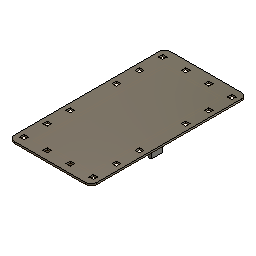
12 V Battery Holder (Autodesk Fusion 360 design; units mm, degrees)
Autodesk Fusion 360 part; units mm, degrees
note: some values were not read from the file. Set by a fixed rule: which sketch regions a step uses.
sketch "Sketch1" plane through (0, 0, 0) normal (0, 1, 0) x (1, 0, 0)
  line L0 (0, 0) -> (58.7375, 0)
  line L1 (58.7375, 0) -> (58.7375, -139.7)
  line L2 (58.7375, -139.7) -> (0, -139.7)
  line L3 (0, -139.7) -> (0, 0)
  line L4 (61.2775, -142.24) -> (-2.54, -142.24)
  line L5 (-2.54, -142.24) -> (-2.54, 2.54)
  line L6 (-2.54, 2.54) -> (61.2775, 2.54)
  line L7 (61.2775, 2.54) -> (61.2775, -142.24)
  line L8 (29.3688, 0) -> (29.3688, -139.7) construction
  line L9 (-8.7313, 6.35) -> (67.4687, 6.35) construction
  line L10 (67.4687, 6.35) -> (67.4688, -146.05)
  line L11 (67.4688, -146.05) -> (-8.7313, -146.05) construction
  line L12 (-8.7313, -146.05) -> (-8.7313, 6.35) construction
  line L13 (-8.7313, 6.35) -> (67.4688, -146.05) construction
  line L14 (67.4687, 6.35) -> (-8.7313, -146.05) construction
  line L15 (-11.1443, 8.763) -> (-6.3183, 8.763)
  line L16 (-6.3183, 8.763) -> (-6.3183, 3.937)
  line L17 (-6.3183, 3.937) -> (-11.1443, 3.937)
  line L18 (-11.1443, 3.937) -> (-11.1443, 8.763)
  line L19 (-11.1443, 8.763) -> (-6.3183, 3.937) construction
  line L20 (-6.3183, 8.763) -> (-11.1443, 3.937) construction
  line L21 (19.0817, 8.763) -> (19.0817, 3.937)
  line L22 (19.0817, 3.937) -> (14.2557, 3.937)
  line L23 (14.2557, 3.937) -> (14.2557, 8.763)
  line L24 (14.2557, 8.763) -> (19.0817, 8.763)
  line L25 (44.4817, 8.763) -> (44.4817, 3.937)
  line L26 (44.4817, 3.937) -> (39.6557, 3.937)
  line L27 (39.6557, 3.937) -> (39.6557, 8.763)
  line L28 (39.6557, 8.763) -> (44.4817, 8.763)
  line L29 (-6.3183, -143.637) -> (-6.3183, -148.463)
  line L30 (-6.3183, -148.463) -> (-11.1443, -148.463)
  line L31 (-11.1443, -148.463) -> (-11.1443, -143.637)
  line L32 (-11.1443, -143.637) -> (-6.3183, -143.637)
  line L33 (19.0817, -143.637) -> (19.0817, -148.463)
  line L34 (19.0817, -148.463) -> (14.2557, -148.463)
  line L35 (14.2557, -148.463) -> (14.2557, -143.637)
  line L36 (14.2557, -143.637) -> (19.0817, -143.637)
  line L37 (44.4817, -143.637) -> (44.4817, -148.463)
  line L38 (44.4817, -148.463) -> (39.6557, -148.463)
  line L39 (39.6557, -148.463) -> (39.6557, -143.637)
  line L40 (39.6557, -143.637) -> (44.4817, -143.637)
  line L41 (69.8817, 8.763) -> (69.8817, 3.937)
  line L42 (69.8817, 3.937) -> (65.0557, 3.937)
  line L43 (65.0557, 3.937) -> (65.0557, 8.763)
  line L44 (65.0557, 8.763) -> (69.8817, 8.763)
  line L45 (69.8817, -143.637) -> (69.8817, -148.463)
  line L46 (69.8817, -148.463) -> (65.0557, -148.463)
  line L47 (65.0557, -148.463) -> (65.0557, -143.637)
  line L48 (65.0557, -143.637) -> (69.8817, -143.637)
  line L49 (74.6125, -155.575) -> (-15.875, -155.575)
  line L50 (-15.875, -155.575) -> (-15.875, 15.875)
  line L51 (-15.875, 15.875) -> (74.6125, 15.875)
  line L52 (74.6125, 15.875) -> (74.6125, -155.575)
  line L53 (58.7375, -125.73) -> (61.2775, -125.73)
  line L54 (61.2775, -125.73) -> (61.2775, -119.38)
  line L55 (61.2775, -119.38) -> (58.7375, -119.38)
  line L56 (58.7375, -119.38) -> (58.7375, -125.73)
  line L57 (60.0075, -125.73) -> (60.0075, -119.38)
  line L58 (29.3688, -69.85) -> (58.7375, -69.85) construction
  line L59 (61.2775, -20.32) -> (58.7375, -20.32)
  line L60 (58.7375, -20.32) -> (58.7375, -13.97)
  line L61 (58.7375, -13.97) -> (61.2775, -13.97)
  line L62 (61.2775, -13.97) -> (61.2775, -20.32)
  line L63 (-11.1443, -21.463) -> (-11.1443, -16.637)
  line L64 (-6.3183, -21.463) -> (-11.1443, -21.463)
  line L65 (-6.3183, -16.637) -> (-6.3183, -21.463)
  line L66 (-11.1443, -16.637) -> (-6.3183, -16.637)
  line L67 (69.8817, -21.463) -> (65.0557, -21.463)
  line L68 (69.8817, -16.637) -> (69.8817, -21.463)
  line L69 (65.0557, -21.463) -> (65.0557, -16.637)
  line L70 (65.0557, -16.637) -> (69.8817, -16.637)
  line L71 (-11.1443, -46.863) -> (-11.1443, -42.037)
  line L72 (-6.3183, -46.863) -> (-11.1443, -46.863)
  line L73 (-6.3183, -42.037) -> (-6.3183, -46.863)
  line L74 (-11.1443, -42.037) -> (-6.3183, -42.037)
  line L75 (69.8817, -46.863) -> (65.0557, -46.863)
  line L76 (69.8817, -42.037) -> (69.8817, -46.863)
  line L77 (65.0557, -46.863) -> (65.0557, -42.037)
  line L78 (65.0557, -42.037) -> (69.8817, -42.037)
  line L79 (-11.1443, -72.263) -> (-11.1443, -67.437)
  line L80 (-6.3183, -72.263) -> (-11.1443, -72.263)
  line L81 (-6.3183, -67.437) -> (-6.3183, -72.263)
  line L82 (-11.1443, -67.437) -> (-6.3183, -67.437)
  line L83 (69.8817, -72.263) -> (65.0557, -72.263)
  line L84 (69.8817, -67.437) -> (69.8817, -72.263)
  line L85 (65.0557, -72.263) -> (65.0557, -67.437)
  line L86 (65.0557, -67.437) -> (69.8817, -67.437)
  line L87 (-11.1443, -97.663) -> (-11.1443, -92.837)
  line L88 (-6.3183, -97.663) -> (-11.1443, -97.663)
  line L89 (-6.3183, -92.837) -> (-6.3183, -97.663)
  line L90 (-11.1443, -92.837) -> (-6.3183, -92.837)
  line L91 (69.8817, -97.663) -> (65.0557, -97.663)
  line L92 (69.8817, -92.837) -> (69.8817, -97.663)
  line L93 (65.0557, -97.663) -> (65.0557, -92.837)
  line L94 (65.0557, -92.837) -> (69.8817, -92.837)
  line L95 (-11.1443, -123.063) -> (-11.1443, -118.237)
  line L96 (-6.3183, -123.063) -> (-11.1443, -123.063)
  line L97 (-6.3183, -118.237) -> (-6.3183, -123.063)
  line L98 (-11.1443, -118.237) -> (-6.3183, -118.237)
  line L99 (69.8817, -123.063) -> (65.0557, -123.063)
  line L100 (69.8817, -118.237) -> (69.8817, -123.063)
  line L101 (65.0557, -123.063) -> (65.0557, -118.237)
  line L102 (65.0557, -118.237) -> (69.8817, -118.237)
  dimension "d1" = 139.7
  dimension "d2" = 58.7375
  dimension "d3" = 2.54
  dimension "d4" = 152.4
  dimension "d5" = 76.2
  dimension "d6" = 4.826
  dimension "d7" = 4.826
  dimension "d10" = 76.2
  dimension "d11" = -152.4
  dimension "d16" = 15.875
  dimension "d27" = 6.35
  dimension "d28" = 17.145
  dimension "d31" = 0
  dimension "d32" = -127
extrude "Extrude1" add sketch "Sketch1" along normal blind 2 contours L0 L1 L2 L3 L4 L5 L6 L7 L53 L61 | L0 L1 L2 L3 L56 L60 | L1 L7 L59 L60 L61 L62 | L1 L7 L55 L59 | L1 L53 L55 L56 L57 | L7 L53 L54 L55 L57 | L10 L83 L84 L86 | L10 L83 L85 L86 | L49 L50 L51 L52 | L79 L80 L81 L82
extrude "Extrude2" add sketch "Sketch1" against normal blind 3.81 contours L0 L1 L2 L3 L4 L5 L6 L7 L53 L61 | L1 L7 L55 L59
sketch "Sketch2" plane through (0, -3.81, 0) normal (0, -1, 0) x (1, 0, 0)
  line L0 (0, 139.7) -> (58.7375, 139.7)
  line L1 (58.7375, 139.7) -> (58.7375, 125.73)
  line L2 (58.7375, 0) -> (0, 0)
  line L3 (0, 0) -> (0, 139.7)
  line L4 (-2.54, -2.54) -> (61.2775, -2.54)
  line L5 (61.2775, 125.73) -> (61.2775, 142.24)
  line L6 (61.2775, 142.24) -> (-2.54, 142.24)
  line L7 (-2.54, 142.24) -> (-2.54, -2.54)
  line L8 (-2.54, 69.85) -> (61.2775, 69.85)
  line L9 (-2.54, 76.2) -> (0, 76.2)
  line L10 (0, 76.2) -> (0, 63.5)
  line L11 (0, 63.5) -> (-2.54, 63.5)
  line L12 (-2.54, 63.5) -> (-2.54, 76.2)
  line L13 (58.7375, 76.2) -> (61.2775, 76.2)
  line L14 (61.2775, 76.2) -> (61.2775, 63.5)
  line L15 (61.2775, 63.5) -> (58.7375, 63.5)
  line L16 (58.7375, 63.5) -> (58.7375, 76.2)
  line L17 (58.7375, 125.73) -> (61.2775, 125.73)
  line L18 (61.2775, -2.54) -> (61.2775, 13.97)
  line L19 (61.2775, 13.97) -> (58.7375, 13.97)
  line L20 (58.7375, 13.97) -> (58.7375, 0)
  line L21 (61.2775, 119.38) -> (61.2775, 20.32)
  dimension "d21" = 12.7
  measures "d21" distance of L2.end
extrude "Extrude3" add sketch "Sketch2" along normal blind 12.065 contours L3 L7 L8 L9 L10 L12 | L3 L7 L8 L10 L11 L12 | L8 L13 L14 L16 L21 | L8 L14 L15 L16 L21
sketch "Sketch3" plane through (0, -15.875, 0) normal (0, -1, 0) x (1, 0, 0)
  line L0 (58.7375, 63.5) -> (61.2775, 63.5)
  line L1 (61.2775, 63.5) -> (61.2775, 76.2)
  line L2 (61.2775, 76.2) -> (58.7375, 76.2)
  line L3 (58.7375, 76.2) -> (58.7375, 63.5)
  line L4 (-2.54, 63.5) -> (0, 63.5)
  line L5 (0, 63.5) -> (0, 76.2)
  line L6 (0, 76.2) -> (-2.54, 76.2)
  line L7 (-2.54, 76.2) -> (-2.54, 63.5)
  line L8 (-2.54, 76.2) -> (2.54, 76.2)
  line L9 (2.54, 76.2) -> (2.54, 63.5)
  line L10 (2.54, 63.5) -> (-2.54, 63.5)
  line L11 (-2.54, 63.5) -> (-2.54, 76.2)
  line L12 (61.2775, 76.2) -> (56.1975, 76.2)
  line L13 (56.1975, 76.2) -> (56.1975, 63.5)
  line L14 (56.1975, 63.5) -> (61.2775, 63.5)
  line L15 (61.2775, 63.5) -> (61.2775, 76.2)
  dimension "d24" = 2.54
extrude "Extrude4" add sketch "Sketch3" along normal blind 3.175
chamfer "Chamfer1" distance 2.54 angle 45 2 edges at (2.54, -19.05, 69.85) (56.1975, -19.05, 69.85)
fillet "Fillet1" radius 6.35 4 edges at (-1.27, -3.81, 63.5) (60.0075, -3.81, 63.5) (60.0075, -3.81, 76.2) (-1.27, -3.81, 76.2)
fillet "Fillet2" radius 6.35 4 edges at (-15.875, 1, -15.875) (74.6125, 1, -15.875) (74.6125, 1, 155.575) (-15.875, 1, 155.575)
sketch "Sketch4" plane through (0, 0, 0) normal (0, -1, 0) x (1, 0, 0)
  line L0 (61.2775, 20.32) -> (58.7375, 20.32)
  line L1 (58.7375, 20.32) -> (58.7375, 119.38)
  line L2 (58.7375, 119.38) -> (61.2775, 119.38)
  line L3 (61.2775, 119.38) -> (61.2775, 20.32)
  line L4 (58.7375, 139.7) -> (0, 139.7)
  line L5 (0, 139.7) -> (0, 0)
  line L6 (0, 0) -> (58.7375, 0)
  line L7 (58.7375, 0) -> (58.7375, 13.97)
  line L8 (58.7375, 13.97) -> (61.2775, 13.97)
  line L9 (61.2775, 13.97) -> (61.2775, -2.54)
  line L10 (61.2775, -2.54) -> (-2.54, -2.54)
  line L11 (-2.54, -2.54) -> (-2.54, 142.24)
  line L12 (-2.54, 142.24) -> (61.2775, 142.24)
  line L13 (61.2775, 142.24) -> (61.2775, 125.73)
  line L14 (61.2775, 125.73) -> (58.7375, 125.73)
  line L15 (58.7375, 125.73) -> (58.7375, 139.7)
  line L16 (65.0557, 42.037) -> (65.0557, 46.863)
  line L17 (65.0557, 46.863) -> (69.8817, 46.863)
  line L18 (69.8817, 46.863) -> (69.8817, 42.037)
  line L19 (69.8817, 42.037) -> (65.0557, 42.037)
  line L20 (65.0557, 16.637) -> (65.0557, 21.463)
  line L21 (65.0557, 21.463) -> (69.8817, 21.463)
  line L22 (69.8817, 21.463) -> (69.8817, 16.637)
  line L23 (69.8817, 16.637) -> (65.0557, 16.637)
  line L24 (65.0557, 92.837) -> (65.0557, 97.663)
  line L25 (65.0557, 97.663) -> (69.8817, 97.663)
  line L26 (69.8817, 97.663) -> (69.8817, 92.837)
  line L27 (69.8817, 92.837) -> (65.0557, 92.837)
  line L28 (65.0557, 118.237) -> (65.0557, 123.063)
  line L29 (65.0557, 123.063) -> (69.8817, 123.063)
  line L30 (69.8817, 123.063) -> (69.8817, 118.237)
  line L31 (69.8817, 118.237) -> (65.0557, 118.237)
  line L32 (65.0557, 143.637) -> (65.0557, 148.463)
  line L33 (65.0557, 148.463) -> (69.8817, 148.463)
  line L34 (69.8817, 148.463) -> (69.8817, 143.637)
  line L35 (69.8817, 143.637) -> (65.0557, 143.637)
  line L36 (65.0557, -8.763) -> (65.0557, -3.937)
  line L37 (65.0557, -3.937) -> (69.8817, -3.937)
  line L38 (69.8817, -3.937) -> (69.8817, -8.763)
  line L39 (69.8817, -8.763) -> (65.0557, -8.763)
  line L40 (-11.1443, 118.237) -> (-11.1443, 123.063)
  line L41 (-11.1443, 123.063) -> (-6.3183, 123.063)
  line L42 (-6.3183, 123.063) -> (-6.3183, 118.237)
  line L43 (-6.3183, 118.237) -> (-11.1443, 118.237)
  line L44 (-11.1443, 92.837) -> (-11.1443, 97.663)
  line L45 (-11.1443, 97.663) -> (-6.3183, 97.663)
  line L46 (-6.3183, 97.663) -> (-6.3183, 92.837)
  line L47 (-6.3183, 92.837) -> (-11.1443, 92.837)
  line L48 (-11.1443, 42.037) -> (-11.1443, 46.863)
  line L49 (-11.1443, 46.863) -> (-6.3183, 46.863)
  line L50 (-6.3183, 46.863) -> (-6.3183, 42.037)
  line L51 (-6.3183, 42.037) -> (-11.1443, 42.037)
  line L52 (-11.1443, 16.637) -> (-11.1443, 21.463)
  line L53 (-11.1443, 21.463) -> (-6.3183, 21.463)
  line L54 (-6.3183, 21.463) -> (-6.3183, 16.637)
  line L55 (-6.3183, 16.637) -> (-11.1443, 16.637)
  line L56 (39.6557, 143.637) -> (39.6557, 148.463)
  line L57 (39.6557, 148.463) -> (44.4817, 148.463)
  line L58 (44.4817, 148.463) -> (44.4817, 143.637)
  line L59 (44.4817, 143.637) -> (39.6557, 143.637)
  line L60 (14.2557, 143.637) -> (14.2557, 148.463)
  line L61 (14.2557, 148.463) -> (19.0817, 148.463)
  line L62 (19.0817, 148.463) -> (19.0817, 143.637)
  line L63 (19.0817, 143.637) -> (14.2557, 143.637)
  line L64 (-11.1443, 143.637) -> (-11.1443, 148.463)
  line L65 (-11.1443, 148.463) -> (-6.3183, 148.463)
  line L66 (-6.3183, 148.463) -> (-6.3183, 143.637)
  line L67 (-6.3183, 143.637) -> (-11.1443, 143.637)
  line L68 (39.6557, -8.763) -> (39.6557, -3.937)
  line L69 (39.6557, -3.937) -> (44.4817, -3.937)
  line L70 (44.4817, -3.937) -> (44.4817, -8.763)
  line L71 (44.4817, -8.763) -> (39.6557, -8.763)
  line L72 (-11.1443, -3.937) -> (-6.3183, -3.937)
  line L73 (-6.3183, -3.937) -> (-6.3183, -8.763)
  line L74 (-6.3183, -8.763) -> (-11.1443, -8.763)
  line L75 (-11.1443, -8.763) -> (-11.1443, -3.937)
  line L76 (14.2557, -8.763) -> (14.2557, -3.937)
  line L77 (14.2557, -3.937) -> (19.0817, -3.937)
  line L78 (19.0817, -3.937) -> (19.0817, -8.763)
  line L79 (19.0817, -8.763) -> (14.2557, -8.763)
  arc A0 (-9.525, 155.575) -> (-15.875, 149.225) centre (-9.525, 149.225) ccw
  line L80 (-15.875, 149.225) -> (-15.875, -9.525)
  arc A1 (-15.875, -9.525) -> (-9.525, -15.875) centre (-9.525, -9.525) ccw
  line L81 (-9.525, -15.875) -> (68.2625, -15.875)
  arc A2 (68.2625, -15.875) -> (74.6125, -9.525) centre (68.2625, -9.525) ccw
  line L82 (74.6125, -9.525) -> (74.6125, 149.225)
  arc A3 (74.6125, 149.225) -> (68.2625, 155.575) centre (68.2625, 149.225) ccw
  line L83 (68.2625, 155.575) -> (-9.525, 155.575)
equation "d22 = 0.625 in - 0.15 in"
